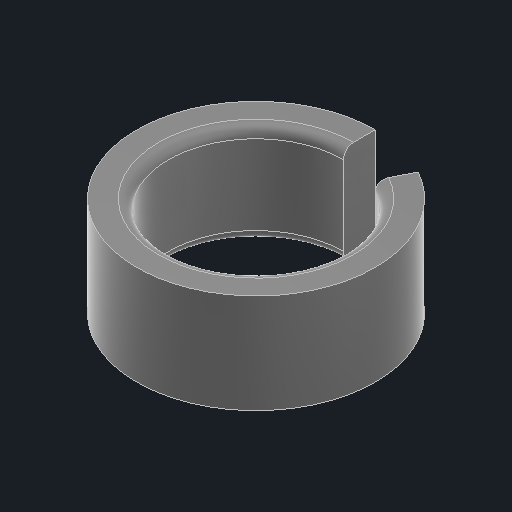
# Autodesk Inventor part: fittingRingInstalled
Saved by Autodesk Inventor 2023 (Build 270158000, 158)
## iProperties
Created: 2023-06-24
Part Number: fittingRingInstalled
Material: Пластик ПАЭК
Document SubType Name: Modeling
Designer: khrip
Density: 1.32 g/cm^3
Appearance: Гладкая — черная
Author: khrip
Autodesk Inventor part; units mm, degrees
ref_plane "YZ Plane" through (0, 0, 0) normal (1, 0, 0) x (0, 1, 0)
ref_plane "XZ Plane" through (0, 0, 0) normal (0, 1, 0) x (-1, 0, 0)
ref_plane "XY Plane" through (0, 0, 0) normal (0, 0, 1) x (1, 0, 0)
sketch "Эскиз1" plane through (0, 0, 0) normal (0, 1, 0) x (-1, 0, 0)
  circle A0 centre (0, 0) radius 6
  circle A1 centre (0, 0) radius 4.4
  dimension "d6" = 12
  dimension "d7" = 8.8
  constraints: 2 centre point, 1 coincident
  measures "d6" diameter of A0
  measures "d7" diameter of A1
extrude "Выдавливание1" add sketch "Эскиз1" along normal blind 5
sketch "Эскиз2" plane through (0, 5, 0) normal (0, 1, 0) x (1, 0, 0)
  circle A0 centre (0, 0) radius 4.4 projected
  arc A1 (2.2, 3.8105) -> (0, 4.4) centre (0, 0) ccw
  line L0 (0, 0) -> (2.2, 3.8105) construction
  line L1 (0, 0) -> (0, 4.4) construction
  line L2 (2.2, 3.8105) -> (3.5243, 6.4533)
  line L3 (0, 4.4) -> (0, 6.8034)
  circle A2 centre (0, 0) radius 6 projected
  point P0 (2.9177, 5.2428)
  point P1 (0, 6)
  dimension "d8" = 30
  constraints: 8 end point, 3 point on circle, 1 centre point, 1 coincident, 1 vertical
  measures "d8" angle of L0 L1
extrude "Выдавливание2" cut sketch "Эскиз2" against normal blind 5 contours A0 L3 A2 L2 picked at (0.3369, 5.4381)
fillet "Сопряжение2" radius 0.5 2 edges at (-1.1388, 0, 4.2501) (-1.1388, 5, 4.2501)
